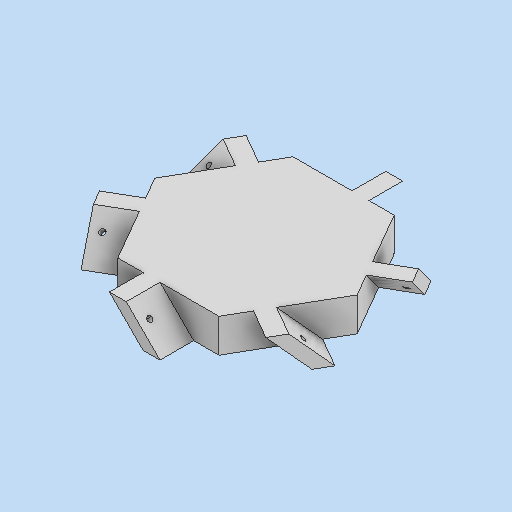
# Autodesk Inventor part: hub
Saved by Autodesk Inventor 2026 (Build 300175000, 175)
## iProperties
Created: 2026-01-30
Part Number: hub
Material: Generic
Document SubType Name: Modeling
Designer: mones
Density: 1 g/cm^3
Appearance: Default
Author: mones
Autodesk Inventor part; units mm, degrees
ref_plane "YZ Plane" through (0, 0, 0) normal (1, 0, 0) x (0, 1, 0)
ref_plane "XZ Plane" through (0, 0, 0) normal (0, 1, 0) x (-1, 0, 0)
ref_plane "XY Plane" through (0, 0, 0) normal (0, 0, 1) x (1, 0, 0)
sketch "Sketch1" plane through (0, 0, 0) normal (0, 1, 0) x (-1, 0, 0)
  circle A0 centre (0, 0) radius 15
  circle A1 centre (0, 0) radius 10
  line L0 (0, 0) -> (-15, 0)
  line L1 (-15, 0) -> (-7.5, 12.9904)
  line L2 (-7.5, 12.9904) -> (0, 0)
  line L3 (-7.5, 12.9904) -> (7.5, 12.9904)
  line L4 (7.5, 12.9904) -> (15, 0)
  line L5 (15, 0) -> (7.5, -12.9904)
  line L6 (7.5, -12.9904) -> (-7.5, -12.9904)
  line L7 (-7.5, -12.9904) -> (-15, 0)
  line L8 (0, 0) -> (7.5, 12.9904)
  line L9 (0, 0) -> (15, 0)
  line L10 (0, 0) -> (7.5, -12.9904)
  line L11 (0, 0) -> (-7.5, -12.9904)
  constraints: 24 end point, 4 horizontal, 1 centre point, 1 coincident, 9 other
extrude "Extrusion3" add sketch "Sketch1" along normal blind 5 contours L7 L0 A1 L11 | L11 A1 L0
sketch "Sketch5" plane through (7.5, 0, -12.9904) normal (0.866, 0, -0.5) x (-0.5, 0, -0.866)
  line L0 (-15, 0) -> (0, 0) projected
  line L1 (0, 0) -> (0, 5) projected
  line L2 (-15, 5) -> (0, 5) projected
  line L3 (-15, 0) -> (-15, 5) projected
  line L4 (0, 0) -> (-15, 5)
  line L5 (-15, 0) -> (0, 5)
  line L6 (-7.5, 2.5) -> (-7.5, 5)
  line L7 (-7.5, 5) -> (-10, 5)
  line L8 (-10, 5) -> (-7.5, 2.5)
  line L9 (-7.5, 2.5) -> (-5, 0)
  line L10 (-10, 5) -> (-8.75, 5)
  line L11 (-8.75, 5) -> (-3.75, 0)
  line L12 (-3.75, 0) -> (-6.25, 0)
  line L13 (-6.25, 0) -> (-11.25, 5)
  line L14 (-10, 5) -> (-11.25, 5)
  dimension "d18" = 2.5
  dimension "d19" = 2.5
  constraints: 22 end point, 6 point on line, 3 midpoint, 3 parallel
  measures "d18" distance of L6.end L7.end
  measures "d19" distance of L11.end L12.end
extrude "Extrusion4" add sketch "Sketch5" along normal blind 5 contours L13 L5 L9 L0 | L13 L4 L5 | L9 L4 L11 L0 | L2 L8 L4 L13 | L5 L11 L4 | L6 L11 L5 | L8 L2 L11 L6
sketch "Sketch6" plane through (11.875, 5, -5.4127) normal (-0.3536, 0.7071, -0.6124) x (0.866, 0, -0.5)
  line L0 (0, 0) -> (0, 7.0711) projected
  line L1 (0, 0) -> (5, 0) projected
  line L2 (5, 7.0711) -> (5, 0) projected
  line L3 (0, 7.0711) -> (5, 7.0711) projected
  line L4 (0, 0) -> (5, 7.0711)
  line L5 (5, 0) -> (0, 7.0711)
  line L6 (2.5, 3.5355) -> (2.5, 2.7855)
  line L7 (2.5, 2.7855) -> (3.5, 2.7855)
  circle A0 centre (3.5, 2.7855) radius 0.4
  point P0 (3.2526, 2.4712)
  point P1 (3.1212, 2.657)
  dimension "d22" = 0.75
  dimension "d26" = 1
  dimension "d27" = 0.8
  constraints: 8 end point, 2 coincident, 1 centre point, 1 horizontal, 1 midpoint, 1 vertical
  measures "d22" distance of L6.start L6.end
  measures "d26" distance of L7.start L7.end
  measures "d27" diameter of A0
extrude "Extrusion5" cut sketch "Sketch6" against normal blind 5 contours L5 A0 picked at (3.3911, 2.7263)
pattern_circular "Circular Pattern1" count 6 over 360 about axis through (0, 0, 0) along (0, 1, 0) of "Extrusion3", "Extrusion4", "Extrusion5"
body "Solid2"
